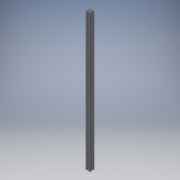
# Autodesk Inventor part: Propile_60
Saved by Autodesk Inventor 2019 (Build 230136000, 136)
## iProperties
Created: 2019-04-05
Part Number: Propile_60
Material: 일반
Document SubType Name: Modeling
Designer: hinmo
Density: 1 g/cm^3
Appearance: 기본값
Author: hinmo
Autodesk Inventor part; units mm, degrees
ref_plane "YZ Plane" through (0, 0, 0) normal (1, 0, 0) x (0, 1, 0)
ref_plane "XZ Plane" through (0, 0, 0) normal (0, 1, 0) x (-1, 0, 0)
ref_plane "XY Plane" through (0, 0, 0) normal (0, 0, 1) x (1, 0, 0)
sketch "스케치1" plane through (0, 0, 0) normal (0, 1, 0) x (-1, 0, 0)
  line L0 (2.65, 8.5) -> (2.65, 10)
  line L1 (9, 10) -> (2.65, 10)
  arc A0 (10, 9) -> (9, 10) centre (9, 9) ccw
  line L2 (10, 2.65) -> (10, 9)
  line L3 (8.5, 2.65) -> (10, 2.65)
  line L4 (8.5, 4.15) -> (8.5, 2.65)
  line L5 (4.9, 4.15) -> (8.5, 4.15)
  arc A1 (4.9, 4.15) -> (4.9, -4.15) centre (9.482, 0) ccw
  line L6 (8.5, -4.15) -> (4.9, -4.15)
  line L7 (8.5, -2.65) -> (8.5, -4.15)
  line L8 (10, -2.65) -> (8.5, -2.65)
  line L9 (10, -9) -> (10, -2.65)
  arc A2 (9, -10) -> (10, -9) centre (9, -9) ccw
  line L10 (2.65, -10) -> (9, -10)
  line L11 (2.65, -10) -> (2.65, -8.5)
  line L12 (2.65, -8.5) -> (4.15, -8.5)
  line L13 (4.15, -8.5) -> (4.15, -4.9)
  arc A3 (4.15, -4.9) -> (-4.15, -4.9) centre (0, -9.482) ccw
  line L14 (-4.15, -4.9) -> (-4.15, -8.5)
  line L15 (-4.15, -8.5) -> (-2.65, -8.5)
  line L16 (-2.65, -8.5) -> (-2.65, -10)
  line L17 (-9, -10) -> (-2.65, -10)
  arc A4 (-10, -9) -> (-9, -10) centre (-9, -9) ccw
  line L18 (-10, -2.65) -> (-10, -9)
  line L19 (-10, -2.65) -> (-8.5, -2.65)
  line L20 (-8.5, -2.65) -> (-8.5, -4.15)
  line L21 (-8.5, -4.15) -> (-4.9, -4.15)
  arc A5 (-4.9, -4.15) -> (-4.9, 4.15) centre (-9.482, 0) ccw
  line L22 (-4.9, 4.15) -> (-8.5, 4.15)
  line L23 (-8.5, 4.15) -> (-8.5, 2.65)
  line L24 (-8.5, 2.65) -> (-10, 2.65)
  line L25 (-10, 9) -> (-10, 2.65)
  arc A6 (-9, 10) -> (-10, 9) centre (-9, 9) ccw
  line L26 (-2.65, 10) -> (-9, 10)
  line L27 (-2.65, 10) -> (-2.65, 8.5)
  line L28 (-2.65, 8.5) -> (-4.15, 8.5)
  line L29 (-4.15, 8.5) -> (-4.15, 4.9)
  arc A7 (-4.15, 4.9) -> (4.15, 4.9) centre (0, 9.482) ccw
  line L30 (4.15, 4.9) -> (4.15, 8.5)
  line L31 (4.15, 8.5) -> (2.65, 8.5)
  circle A8 centre (-7, 7) radius 2
  circle A9 centre (7, 7) radius 2
  circle A10 centre (0, 0) radius 2.15
  circle A11 centre (-7, -7) radius 2
  circle A12 centre (7, -7) radius 2
  constraints: 64 end point, 16 point on circle, 13 centre point
extrude "돌출1" add sketch "스케치1" along normal blind 600
